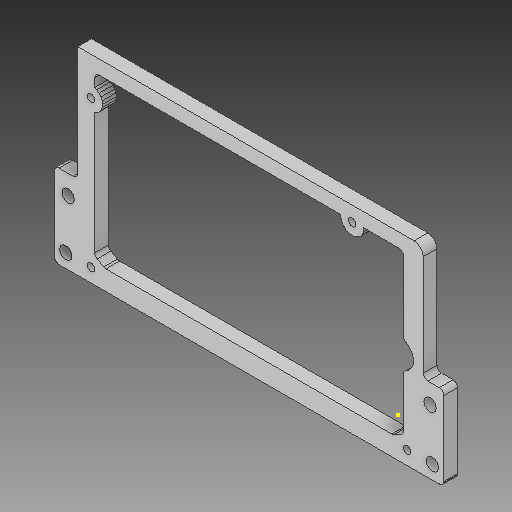
# Autodesk Inventor part: PSU Mount Hipro
Saved by Autodesk Inventor 2018 (Build 220112000, 112)
## iProperties
Created: 2016-07-03
Part Number: PSU Mount Hipro
Material: Generic
Document SubType Name: Modeling
Designer: joshm
Density: 1 g/cm^3
Appearance: Default
Author: joshm
Autodesk Inventor part; units mm, degrees
(part 1 of 2)
ref_plane "YZ Plane" through (0, 0, 0) normal (1, 0, 0) x (0, 1, 0)
ref_plane "XZ Plane" through (0, 0, 0) normal (0, 1, 0) x (-1, 0, 0)
ref_plane "XY Plane" through (0, 0, 0) normal (0, 0, 1) x (1, 0, 0)
sketch "Sketch1" plane through (0, 0, 0) normal (0, 0, 1) x (1, 0, 0)
  line L0 (-149.9319, 87.3176) -> (-150, 86.8)
  line L1 (-150, 86.8) -> (-150, -15.2)
  line L2 (-150, -15.2) -> (-149.9319, -15.7176)
  line L3 (-149.9319, -15.7176) -> (-149.8478, -15.9654)
  line L4 (-149.8478, -15.9654) -> (-149.7321, -16.2)
  line L5 (-149.7321, -16.2) -> (-149.5867, -16.4175)
  line L6 (-149.5867, -16.4175) -> (-149.4142, -16.6142)
  line L7 (-149.4142, -16.6142) -> (-149.2175, -16.7867)
  line L8 (-149.2175, -16.7867) -> (-149, -16.9321)
  line L9 (-149, -16.9321) -> (-148.7654, -17.0478)
  line L10 (-148.7654, -17.0478) -> (-148.5176, -17.1319)
  line L11 (-148.5176, -17.1319) -> (-148, -17.2)
  line L12 (-148, -17.2) -> (18, -17.2)
  line L13 (18, -17.2) -> (18.5176, -17.1319)
  line L14 (18.5176, -17.1319) -> (18.7654, -17.0478)
  line L15 (18.7654, -17.0478) -> (19, -16.9321)
  line L16 (19, -16.9321) -> (19.2175, -16.7867)
  line L17 (19.2175, -16.7867) -> (19.4142, -16.6142)
  line L18 (19.4142, -16.6142) -> (19.5867, -16.4175)
  line L19 (19.5867, -16.4175) -> (19.7321, -16.2)
  line L20 (19.7321, -16.2) -> (19.8478, -15.9654)
  line L21 (19.8478, -15.9654) -> (19.9319, -15.7176)
  line L22 (19.9319, -15.7176) -> (20, -15.2)
  line L23 (20, -15.2) -> (20, 19.2664)
  line L24 (20, 19.2664) -> (11, 19.2664)
  line L25 (11, 19.2664) -> (11, 88.8)
  line L26 (11, 88.8) -> (-148, 88.8)
  line L27 (-148, 88.8) -> (-148.5176, 88.7319)
  line L28 (-148.5176, 88.7319) -> (-148.7654, 88.6478)
  line L29 (-148.7654, 88.6478) -> (-149, 88.5321)
  line L30 (-149, 88.5321) -> (-149.2175, 88.3867)
  line L31 (-149.2175, 88.3867) -> (-149.4142, 88.2142)
  line L32 (-149.4142, 88.2142) -> (-149.5867, 88.0175)
  line L33 (-149.5867, 88.0175) -> (-149.7321, 87.8)
  line L34 (-149.7321, 87.8) -> (-149.8478, 87.5654)
  line L35 (-149.8478, 87.5654) -> (-149.9319, 87.3176)
  line L36 (14.6729, 8.2886) -> (14, 8.2)
  line L37 (14, 8.2) -> (13.3271, 8.2886)
  line L38 (13.3271, 8.2886) -> (12.7, 8.5483)
  line L39 (12.7, 8.5483) -> (12.1615, 8.9615)
  line L40 (12.1615, 8.9615) -> (11.7483, 9.5)
  line L41 (11.7483, 9.5) -> (11.4886, 10.1271)
  line L42 (11.4886, 10.1271) -> (11.4, 10.8)
  line L43 (11.4, 10.8) -> (11.4886, 11.4729)
  line L44 (11.4886, 11.4729) -> (11.7483, 12.1)
  line L45 (11.7483, 12.1) -> (12.1615, 12.6385)
  line L46 (12.1615, 12.6385) -> (12.7, 13.0517)
  line L47 (12.7, 13.0517) -> (13.3271, 13.3114)
  line L48 (13.3271, 13.3114) -> (14, 13.4)
  line L49 (14, 13.4) -> (14.6729, 13.3114)
  line L50 (14.6729, 13.3114) -> (15.3, 13.0517)
  line L51 (15.3, 13.0517) -> (15.8385, 12.6385)
  line L52 (15.8385, 12.6385) -> (16.2517, 12.1)
  line L53 (16.2517, 12.1) -> (16.5114, 11.4729)
  line L54 (16.5114, 11.4729) -> (16.6, 10.8)
  line L55 (16.6, 10.8) -> (16.5114, 10.1271)
  line L56 (16.5114, 10.1271) -> (16.2517, 9.5)
  line L57 (16.2517, 9.5) -> (15.8385, 8.9615)
  line L58 (15.8385, 8.9615) -> (15.3, 8.5483)
  line L59 (15.3, 8.5483) -> (14.6729, 8.2886)
  line L60 (-135.5455, -11.6141) -> (-135.6, -11.2)
  line L61 (-135.6, -11.2) -> (-135.5455, -10.7859)
  line L62 (-135.5455, -10.7859) -> (-135.3856, -10.4)
  line L63 (-135.3856, -10.4) -> (-135.1314, -10.0686)
  line L64 (-135.1314, -10.0686) -> (-134.8, -9.8144)
  line L65 (-134.8, -9.8144) -> (-134.4141, -9.6545)
  line L66 (-134.4141, -9.6545) -> (-134, -9.6)
  line L67 (-134, -9.6) -> (-133.5859, -9.6545)
  line L68 (-133.5859, -9.6545) -> (-133.2, -9.8144)
  line L69 (-133.2, -9.8144) -> (-132.8686, -10.0686)
  line L70 (-132.8686, -10.0686) -> (-132.6144, -10.4)
  line L71 (-132.6144, -10.4) -> (-132.4545, -10.7859)
  line L72 (-132.4545, -10.7859) -> (-132.4, -11.2)
  line L73 (-132.4, -11.2) -> (-132.4545, -11.6141)
  line L74 (-132.4545, -11.6141) -> (-132.6144, -12)
  line L75 (-132.6144, -12) -> (-132.8686, -12.3314)
  line L76 (-132.8686, -12.3314) -> (-133.2, -12.5856)
  line L77 (-133.2, -12.5856) -> (-133.5859, -12.7455)
  line L78 (-133.5859, -12.7455) -> (-134, -12.8)
  line L79 (-134, -12.8) -> (-134.4141, -12.7455)
  line L80 (-134.4141, -12.7455) -> (-134.8, -12.5856)
  line L81 (-134.8, -12.5856) -> (-135.1314, -12.3314)
  line L82 (-135.1314, -12.3314) -> (-135.3856, -12)
  line L83 (-135.3856, -12) -> (-135.5455, -11.6141)
  line L84 (5.6, -11.2) -> (5.5455, -11.6141)
  line L85 (5.5455, -11.6141) -> (5.3856, -12)
  line L86 (5.3856, -12) -> (5.1314, -12.3314)
  line L87 (5.1314, -12.3314) -> (4.8, -12.5856)
  line L88 (4.8, -12.5856) -> (4.4141, -12.7455)
  line L89 (4.4141, -12.7455) -> (4, -12.8)
  line L90 (4, -12.8) -> (3.5859, -12.7455)
  line L91 (3.5859, -12.7455) -> (3.2, -12.5856)
  line L92 (3.2, -12.5856) -> (2.8686, -12.3314)
  line L93 (2.8686, -12.3314) -> (2.6144, -12)
  line L94 (2.6144, -12) -> (2.4545, -11.6141)
  line L95 (2.4545, -11.6141) -> (2.4, -11.2)
  line L96 (2.4, -11.2) -> (2.4545, -10.7859)
  line L97 (2.4545, -10.7859) -> (2.6144, -10.4)
  line L98 (2.6144, -10.4) -> (2.8686, -10.0686)
  line L99 (2.8686, -10.0686) -> (3.2, -9.8144)
  line L100 (3.2, -9.8144) -> (3.5859, -9.6545)
  line L101 (3.5859, -9.6545) -> (4, -9.6)
  line L102 (4, -9.6) -> (4.4141, -9.6545)
  line L103 (4.4141, -9.6545) -> (4.8, -9.8144)
  line L104 (4.8, -9.8144) -> (5.1314, -10.0686)
  line L105 (5.1314, -10.0686) -> (5.3856, -10.4)
  line L106 (5.3856, -10.4) -> (5.5455, -10.7859)
  line L107 (5.5455, -10.7859) -> (5.6, -11.2)
  line L108 (-108.7, 78.5483) -> (-109.3271, 78.2886)
  line L109 (-109.3271, 78.2886) -> (-110, 78.2)
  line L110 (-110, 78.2) -> (-110.6729, 78.2886)
  line L111 (-110.6729, 78.2886) -> (-111.3, 78.5483)
  line L112 (-111.3, 78.5483) -> (-111.8385, 78.9615)
  line L113 (-111.8385, 78.9615) -> (-112.2517, 79.5)
  line L114 (-112.2517, 79.5) -> (-112.5114, 80.1271)
  line L115 (-112.5114, 80.1271) -> (-112.6, 80.8)
  line L116 (-112.6, 80.8) -> (-112.5114, 81.4729)
  line L117 (-112.5114, 81.4729) -> (-112.2517, 82.1)
  line L118 (-112.2517, 82.1) -> (-111.8385, 82.6385)
  line L119 (-111.8385, 82.6385) -> (-111.3, 83.0517)
  line L120 (-111.3, 83.0517) -> (-110.6729, 83.3114)
  line L121 (-110.6729, 83.3114) -> (-110, 83.4)
  line L122 (-110, 83.4) -> (-109.3271, 83.3114)
  line L123 (-109.3271, 83.3114) -> (-108.7, 83.0517)
  line L124 (-108.7, 83.0517) -> (-108.1615, 82.6385)
  line L125 (-108.1615, 82.6385) -> (-107.7483, 82.1)
  line L126 (-107.7483, 82.1) -> (-107.4886, 81.4729)
  line L127 (-107.4886, 81.4729) -> (-107.4, 80.8)
  line L128 (-107.4, 80.8) -> (-107.4886, 80.1271)
  line L129 (-107.4886, 80.1271) -> (-107.7483, 79.5)
  line L130 (-107.7483, 79.5) -> (-108.1615, 78.9615)
  line L131 (-108.1615, 78.9615) -> (-108.7, 78.5483)
  line L132 (-142.8159, -4.2) -> (-142.8159, -7.2)
  line L133 (-142.8159, -7.2) -> (-147.8159, -7.2)
  line L134 (-147.8159, -7.2) -> (-147.8159, -4.2)
  line L135 (-147.8159, -4.2) -> (-142.8159, -4.2)
  line L136 (-18.8686, 61.6686) -> (-19.2, 61.4144)
  line L137 (-19.2, 61.4144) -> (-19.5859, 61.2545)
  line L138 (-19.5859, 61.2545) -> (-20, 61.2)
  line L139 (-20, 61.2) -> (-20.4141, 61.2545)
  line L140 (-20.4141, 61.2545) -> (-20.8, 61.4144)
  line L141 (-20.8, 61.4144) -> (-21.1314, 61.6686)
  line L142 (-21.1314, 61.6686) -> (-21.3856, 62)
  line L143 (-21.3856, 62) -> (-21.5455, 62.3859)
  line L144 (-21.5455, 62.3859) -> (-21.6, 62.8)
  line L145 (-21.6, 62.8) -> (-21.5455, 63.2141)
  line L146 (-21.5455, 63.2141) -> (-21.3856, 63.6)
  line L147 (-21.3856, 63.6) -> (-21.1314, 63.9314)
  line L148 (-21.1314, 63.9314) -> (-20.8, 64.1856)
  line L149 (-20.8, 64.1856) -> (-20.4141, 64.3455)
  line L150 (-20.4141, 64.3455) -> (-20, 64.4)
  line L151 (-20, 64.4) -> (-19.5859, 64.3455)
  line L152 (-19.5859, 64.3455) -> (-19.2, 64.1856)
  line L153 (-19.2, 64.1856) -> (-18.8686, 63.9314)
  line L154 (-18.8686, 63.9314) -> (-18.6144, 63.6)
  line L155 (-18.6144, 63.6) -> (-18.4545, 63.2141)
  line L156 (-18.4545, 63.2141) -> (-18.4, 62.8)
  line L157 (-18.4, 62.8) -> (-18.4545, 62.3859)
  line L158 (-18.4545, 62.3859) -> (-18.6144, 62)
  line L159 (-18.6144, 62) -> (-18.8686, 61.6686)
  line L160 (-20, 78.2) -> (-20.6729, 78.2886)
  line L161 (-20.6729, 78.2886) -> (-21.3, 78.5483)
  line L162 (-21.3, 78.5483) -> (-21.8385, 78.9615)
  line L163 (-21.8385, 78.9615) -> (-22.2517, 79.5)
  line L164 (-22.2517, 79.5) -> (-22.5114, 80.1271)
  line L165 (-22.5114, 80.1271) -> (-22.6, 80.8)
  line L166 (-22.6, 80.8) -> (-22.5114, 81.4729)
  line L167 (-22.5114, 81.4729) -> (-22.2517, 82.1)
  line L168 (-22.2517, 82.1) -> (-21.8385, 82.6385)
  line L169 (-21.8385, 82.6385) -> (-21.3, 83.0517)
  line L170 (-21.3, 83.0517) -> (-20.6729, 83.3114)
  line L171 (-20.6729, 83.3114) -> (-20, 83.4)
  line L172 (-20, 83.4) -> (-19.3271, 83.3114)
  line L173 (-19.3271, 83.3114) -> (-18.7, 83.0517)
  line L174 (-18.7, 83.0517) -> (-18.1615, 82.6385)
  line L175 (-18.1615, 82.6385) -> (-17.7483, 82.1)
  line L176 (-17.7483, 82.1) -> (-17.4886, 81.4729)
  line L177 (-17.4886, 81.4729) -> (-17.4, 80.8)
  line L178 (-17.4, 80.8) -> (-17.4886, 80.1271)
  line L179 (-17.4886, 80.1271) -> (-17.7483, 79.5)
  line L180 (-17.7483, 79.5) -> (-18.1615, 78.9615)
  line L181 (-18.1615, 78.9615) -> (-18.7, 78.5483)
  line L182 (-18.7, 78.5483) -> (-19.3271, 78.2886)
  line L183 (-19.3271, 78.2886) -> (-20, 78.2)
  line L184 (-132.4545, 52.3859) -> (-132.6144, 52)
  line L185 (-132.6144, 52) -> (-132.8686, 51.6686)
  line L186 (-132.8686, 51.6686) -> (-133.2, 51.4144)
  line L187 (-133.2, 51.4144) -> (-133.5859, 51.2545)
  line L188 (-133.5859, 51.2545) -> (-134, 51.2)
  line L189 (-134, 51.2) -> (-134.4141, 51.2545)
  line L190 (-134.4141, 51.2545) -> (-134.8, 51.4144)
  line L191 (-134.8, 51.4144) -> (-135.1314, 51.6686)
  line L192 (-135.1314, 51.6686) -> (-135.3856, 52)
  line L193 (-135.3856, 52) -> (-135.5455, 52.3859)
  line L194 (-135.5455, 52.3859) -> (-135.6, 52.8)
  line L195 (-135.6, 52.8) -> (-135.5455, 53.2141)
  line L196 (-135.5455, 53.2141) -> (-135.3856, 53.6)
  line L197 (-135.3856, 53.6) -> (-135.1314, 53.9314)
  line L198 (-135.1314, 53.9314) -> (-134.8, 54.1856)
  line L199 (-134.8, 54.1856) -> (-134.4141, 54.3455)
  line L200 (-134.4141, 54.3455) -> (-134, 54.4)
  line L201 (-134, 54.4) -> (-133.5859, 54.3455)
  line L202 (-133.5859, 54.3455) -> (-133.2, 54.1856)
  line L203 (-133.2, 54.1856) -> (-132.8686, 53.9314)
  line L204 (-132.8686, 53.9314) -> (-132.6144, 53.6)
  line L205 (-132.6144, 53.6) -> (-132.4545, 53.2141)
  line L206 (-132.4545, 53.2141) -> (-132.4, 52.8)
  line L207 (-132.4, 52.8) -> (-132.4545, 52.3859)
  line L208 (-129.6699, 50.3) -> (-129.1704, 51.5059)
  line L209 (-129.1704, 51.5059) -> (-129, 52.8)
  line L210 (-129, 52.8) -> (-129.1704, 54.0941)
  line L211 (-129.1704, 54.0941) -> (-129.6699, 55.3)
  line L212 (-129.6699, 55.3) -> (-130.4645, 56.3355)
  line L213 (-130.4645, 56.3355) -> (-131.5, 57.1301)
  line L214 (-131.5, 57.1301) -> (-132.4, 57.5029)
  line L215 (-132.4, 57.5029) -> (-132.4, 63.2)
  line L216 (-132.4, 63.2) -> (-24.9458, 63.212)
  line L217 (-24.9458, 63.212) -> (-25, 62.8)
  line L218 (-25, 62.8) -> (-24.8296, 61.5059)
  line L219 (-24.8296, 61.5059) -> (-24.3301, 60.3)
  line L220 (-24.3301, 60.3) -> (-23.5355, 59.2645)
  line L221 (-23.5355, 59.2645) -> (-22.5, 58.4699)
  line L222 (-22.5, 58.4699) -> (-21.2941, 57.9704)
  line L223 (-21.2941, 57.9704) -> (-20, 57.8)
  line L224 (-20, 57.8) -> (-18.7059, 57.9704)
  line L225 (-18.7059, 57.9704) -> (-17.5, 58.4699)
  line L226 (-17.5, 58.4699) -> (-16.4645, 59.2645)
  line L227 (-16.4645, 59.2645) -> (-15.6699, 60.3)
  line L228 (-15.6699, 60.3) -> (-15.1704, 61.5059)
  line L229 (-15.1704, 61.5059) -> (-15, 62.8)
  line L230 (-15, 62.8) -> (-15.0542, 63.2118)
  line L231 (-15.0542, 63.2118) -> (2.4, 63.2)
  line L232 (2.4, 63.2) -> (2.4, -6.2)
  line L233 (2.4, -6.2) -> (-2.1698, -8.6089)
  line L234 (-2.1698, -8.6089) -> (-128.0185, -8.6089)
  line L235 (-128.0185, -8.6089) -> (-132.4, -6.2)
  line L236 (-132.4, -6.2) -> (-132.4, 48.0971)
  line L237 (-132.4, 48.0971) -> (-131.5, 48.4699)
  line L238 (-131.5, 48.4699) -> (-130.4645, 49.2645)
  line L239 (-130.4645, 49.2645) -> (-129.6699, 50.3)
  line L240 (-142.392, -10.5012) -> (-142.3, -11.2)
  line L241 (-142.3, -11.2) -> (-142.392, -11.8988)
  line L242 (-142.392, -11.8988) -> (-142.6617, -12.55)
  line L243 (-142.6617, -12.55) -> (-143.0908, -13.1092)
  line L244 (-143.0908, -13.1092) -> (-143.65, -13.5383)
  line L245 (-143.65, -13.5383) -> (-144.3012, -13.808)
  line L246 (-144.3012, -13.808) -> (-145, -13.9)
  line L247 (-145, -13.9) -> (-145.6988, -13.808)
  line L248 (-145.6988, -13.808) -> (-146.35, -13.5383)
  line L249 (-146.35, -13.5383) -> (-146.9092, -13.1092)
  line L250 (-146.9092, -13.1092) -> (-147.3383, -12.55)
  line L251 (-147.3383, -12.55) -> (-147.608, -11.8988)
  line L252 (-147.608, -11.8988) -> (-147.7, -11.2)
  line L253 (-147.7, -11.2) -> (-147.608, -10.5012)
  line L254 (-147.608, -10.5012) -> (-147.3383, -9.85)
  line L255 (-147.3383, -9.85) -> (-146.9092, -9.2908)
  line L256 (-146.9092, -9.2908) -> (-146.35, -8.8617)
  line L257 (-146.35, -8.8617) -> (-145.6988, -8.592)
  line L258 (-145.6988, -8.592) -> (-145, -8.5)
  line L259 (-145, -8.5) -> (-144.3012, -8.592)
  line L260 (-144.3012, -8.592) -> (-143.65, -8.8617)
  line L261 (-143.65, -8.8617) -> (-143.0908, -9.2908)
  line L262 (-143.0908, -9.2908) -> (-142.6617, -9.85)
  line L263 (-142.6617, -9.85) -> (-142.392, -10.5012)
  line L264 (12.3, -11.2) -> (12.392, -10.5012)
  line L265 (12.392, -10.5012) -> (12.6617, -9.85)
  line L266 (12.6617, -9.85) -> (13.0908, -9.2908)
  line L267 (13.0908, -9.2908) -> (13.65, -8.8617)
  line L268 (13.65, -8.8617) -> (14.3012, -8.592)
  line L269 (14.3012, -8.592) -> (15, -8.5)
  line L270 (15, -8.5) -> (15.6988, -8.592)
  line L271 (15.6988, -8.592) -> (16.35, -8.8617)
  line L272 (16.35, -8.8617) -> (16.9092, -9.2908)
  line L273 (16.9092, -9.2908) -> (17.3383, -9.85)
  line L274 (17.3383, -9.85) -> (17.608, -10.5012)
  line L275 (17.608, -10.5012) -> (17.7, -11.2)
  line L276 (17.7, -11.2) -> (17.608, -11.8988)
  line L277 (17.608, -11.8988) -> (17.3383, -12.55)
  line L278 (17.3383, -12.55) -> (16.9092, -13.1092)
  line L279 (16.9092, -13.1092) -> (16.35, -13.5383)
  line L280 (16.35, -13.5383) -> (15.6988, -13.808)
  line L281 (15.6988, -13.808) -> (15, -13.9)
  line L282 (15, -13.9) -> (14.3012, -13.808)
  line L283 (14.3012, -13.808) -> (13.65, -13.5383)
  line L284 (13.65, -13.5383) -> (13.0908, -13.1092)
  line L285 (13.0908, -13.1092) -> (12.6617, -12.55)
  line L286 (12.6617, -12.55) -> (12.392, -11.8988)
  line L287 (12.392, -11.8988) -> (12.3, -11.2)
  line L288 (-142.392, 59.4988) -> (-142.3, 58.8)
  line L289 (-142.3, 58.8) -> (-142.392, 58.1012)
  line L290 (-142.392, 58.1012) -> (-142.6617, 57.45)
  line L291 (-142.6617, 57.45) -> (-143.0908, 56.8908)
  line L292 (-143.0908, 56.8908) -> (-143.65, 56.4617)
  line L293 (-143.65, 56.4617) -> (-144.3012, 56.192)
  line L294 (-144.3012, 56.192) -> (-145, 56.1)
  line L295 (-145, 56.1) -> (-145.6988, 56.192)
  line L296 (-145.6988, 56.192) -> (-146.35, 56.4617)
  line L297 (-146.35, 56.4617) -> (-146.9092, 56.8908)
  line L298 (-146.9092, 56.8908) -> (-147.3383, 57.45)
  line L299 (-147.3383, 57.45) -> (-147.608, 58.1012)
  line L300 (-147.608, 58.1012) -> (-147.7, 58.8)
  line L301 (-147.7, 58.8) -> (-147.608, 59.4988)
  line L302 (-147.608, 59.4988) -> (-147.3383, 60.15)
  line L303 (-147.3383, 60.15) -> (-146.9092, 60.7092)
  line L304 (-146.9092, 60.7092) -> (-146.35, 61.1383)
  line L305 (-146.35, 61.1383) -> (-145.6988, 61.408)
  line L306 (-145.6988, 61.408) -> (-145, 61.5)
  line L307 (-145, 61.5) -> (-144.3012, 61.408)
  line L308 (-144.3012, 61.408) -> (-143.65, 61.1383)
  line L309 (-143.65, 61.1383) -> (-143.0908, 60.7092)
  line L310 (-143.0908, 60.7092) -> (-142.6617, 60.15)
  line L311 (-142.6617, 60.15) -> (-142.392, 59.4988)
  line L312 (-142.1615, 8.9615) -> (-142.3, 8.8553)
  line L313 (-142.3, 8.8553) -> (-142.7, 8.5483)
  line L314 (-142.7, 8.5483) -> (-143.3271, 8.2886)
  line L315 (-143.3271, 8.2886) -> (-144, 8.2)
  line L316 (-144, 8.2) -> (-144.6729, 8.2886)
  line L317 (-144.6729, 8.2886) -> (-145.3, 8.5483)
  line L318 (-145.3, 8.5483) -> (-145.8385, 8.9615)
  line L319 (-145.8385, 8.9615) -> (-146.2517, 9.5)
  line L320 (-146.2517, 9.5) -> (-146.5114, 10.1271)
  line L321 (-146.5114, 10.1271) -> (-146.6, 10.8)
  line L322 (-146.6, 10.8) -> (-146.5114, 11.4729)
  line L323 (-146.5114, 11.4729) -> (-146.2517, 12.1)
  line L324 (-146.2517, 12.1) -> (-145.8385, 12.6385)
  line L325 (-145.8385, 12.6385) -> (-145.3, 13.0517)
  line L326 (-145.3, 13.0517) -> (-144.6729, 13.3114)
  line L327 (-144.6729, 13.3114) -> (-144, 13.4)
  line L328 (-144, 13.4) -> (-143.3271, 13.3114)
  line L329 (-143.3271, 13.3114) -> (-142.7, 13.0517)
  line L330 (-142.7, 13.0517) -> (-142.3, 12.7447)
  line L331 (-142.3, 12.7447) -> (-142.1615, 12.6385)
  line L332 (-142.1615, 12.6385) -> (-141.7483, 12.1)
  line L333 (-141.7483, 12.1) -> (-141.4886, 11.4729)
  line L334 (-141.4886, 11.4729) -> (-141.4, 10.8)
  line L335 (-141.4, 10.8) -> (-141.4886, 10.1271)
  line L336 (-141.4886, 10.1271) -> (-141.7483, 9.5)
  line L337 (-141.7483, 9.5) -> (-142.1615, 8.9615)
  point P0 (0, 0)
  constraints: 676 end point
extrude "Extrusion1" add sketch "Sketch1" along normal blind 6
sketch "Sketch2" plane through (0, 0, 6) normal (0, 0, 1) x (1, 0, 0)
  line L0 (11, 19.2664) -> (11, 88.8) projected
  line L1 (11, 19.2664) -> (11, 24.0664)
  line L2 (11, 19.2664) -> (15.8, 19.2664) construction
  circle A0 centre (11, 24.0664) radius 3
  point P0 (0, 0)
  dimension "d3" = 90
  constraints: 4 end point, 1 centre point, 1 coincident, 1 collinear, 1 horizontal, 1 perpendicular
  measures "d3" angle of L2 L1
extrude "Extrusion2" cut sketch "Sketch2" against normal blind 6
fillet "Fillet1" radius 2 3 edges at (11, 19.2664, 3) (11, 27.0664, 3) (11, 21.0664, 3)
fillet "Fillet2" radius 2 1 edges at (11, 88.8, 3)
fillet "Fillet3" radius 2 3 edges at (-132.4, 63.2, 3) (-132.4, -6.2, 3) (-128.0185, -8.6089, 3)
fillet "Fillet4" radius 2 3 edges at (2.4, 63.2, 3) (-2.1698, -8.6089, 3) (2.4, -6.2, 3)
fillet "Fillet5" radius 2 1 edges at (20, 19.2664, 3)
sketch "Sketch3" plane through (0, 0, 6) normal (0, 0, 1) x (1, 0, 0)
  arc A0 (20, 17.2664) -> (18, 19.2664) centre (18, 17.2664) ccw
  line L0 (18, 19.2664) -> (12.5808, 19.2664)
  arc A1 (10.7904, 20.3751) -> (12.5808, 19.2664) centre (12.5808, 21.2664) ccw
  arc A2 (10.7904, 20.3751) -> (9.8, 21.3169) centre (9, 19.4838) ccw
  arc A3 (9.8, 26.816) -> (9.8, 21.3169) centre (11, 24.0664) ccw
  arc A4 (9.8, 26.816) -> (11, 28.649) centre (9, 28.649) ccw
  line L1 (11, 28.649) -> (11, 86.8) projected
  arc A5 (9, 88.8) -> (11, 86.8) centre (9, 86.8) ccw projected
  line L2 (9, 88.8) -> (-148, 88.8) projected
  line L3 (-148, 88.8) -> (-148.5176, 88.7319) projected
  line L4 (-148.5176, 88.7319) -> (-148.7654, 88.6478) projected
  line L5 (-148.7654, 88.6478) -> (-149, 88.5321) projected
  line L6 (-149, 88.5321) -> (-149.2175, 88.3867) projected
  line L7 (-149.2175, 88.3867) -> (-149.4142, 88.2142) projected
  line L8 (-149.4142, 88.2142) -> (-149.5867, 88.0175) projected
  line L9 (-149.5867, 88.0175) -> (-149.7321, 87.8) projected
  line L10 (-149.7321, 87.8) -> (-149.8478, 87.5654) projected
  line L11 (-149.8478, 87.5654) -> (-149.9319, 87.3176) projected
  line L12 (-149.9319, 87.3176) -> (-150, 86.8) projected
  line L13 (-150, 86.8) -> (-150, -15.2) projected
  line L14 (-150, -15.2) -> (-149.9319, -15.7176) projected
  line L15 (-149.9319, -15.7176) -> (-149.8478, -15.9654) projected
  line L16 (-149.8478, -15.9654) -> (-149.7321, -16.2) projected
  line L17 (-149.7321, -16.2) -> (-149.5867, -16.4175) projected
  line L18 (-149.5867, -16.4175) -> (-149.4142, -16.6142) projected
  line L19 (-149.4142, -16.6142) -> (-149.2175, -16.7867) projected
  line L20 (-149.2175, -16.7867) -> (-149, -16.9321) projected
  line L21 (-149, -16.9321) -> (-148.7654, -17.0478) projected
  line L22 (-148.7654, -17.0478) -> (-148.5176, -17.1319) projected
  line L23 (-148.5176, -17.1319) -> (-148, -17.2) projected
  line L24 (-148, -17.2) -> (18, -17.2) projected
  line L25 (18, -17.2) -> (18.5176, -17.1319) projected
  line L26 (18.5176, -17.1319) -> (18.7654, -17.0478) projected
  line L27 (18.7654, -17.0478) -> (19, -16.9321) projected
  line L28 (19, -16.9321) -> (19.2175, -16.7867) projected
  line L29 (19.2175, -16.7867) -> (19.4142, -16.6142) projected
  line L30 (19.4142, -16.6142) -> (19.5867, -16.4175) projected
  line L31 (19.5867, -16.4175) -> (19.7321, -16.2) projected
  line L32 (19.7321, -16.2) -> (19.8478, -15.9654) projected
  line L33 (19.8478, -15.9654) -> (19.9319, -15.7176) projected
  line L34 (19.9319, -15.7176) -> (20, -15.2) projected
  line L35 (20, -15.2) -> (20, 17.2664) projected
  line L36 (-129, 52.8) -> (-129.1704, 54.0941) projected
  line L37 (-129.1704, 54.0941) -> (-129.6699, 55.3) projected
  line L38 (-129.6699, 55.3) -> (-130.4645, 56.3355) projected
  line L39 (-130.4645, 56.3355) -> (-131.5, 57.1301) projected
  line L40 (-131.5, 57.1301) -> (-132.4, 57.5029) projected
  line L41 (-132.4, 57.5029) -> (-132.4, 61.2002) projected
  arc A6 (-130.4002, 63.2002) -> (-132.4, 61.2002) centre (-130.4, 61.2002) ccw projected
  line L42 (-130.4002, 63.2002) -> (-24.9458, 63.212) projected
  line L43 (-24.9458, 63.212) -> (-25, 62.8) projected
  line L44 (-25, 62.8) -> (-24.8296, 61.5059) projected
  line L45 (-24.8296, 61.5059) -> (-24.3301, 60.3) projected
  line L46 (-24.3301, 60.3) -> (-23.5355, 59.2645) projected
  line L47 (-23.5355, 59.2645) -> (-22.5, 58.4699) projected
  line L48 (-22.5, 58.4699) -> (-21.2941, 57.9704) projected
  line L49 (-21.2941, 57.9704) -> (-20, 57.8) projected
  line L50 (-20, 57.8) -> (-18.7059, 57.9704) projected
  line L51 (-18.7059, 57.9704) -> (-17.5, 58.4699) projected
  line L52 (-17.5, 58.4699) -> (-16.4645, 59.2645) projected
  line L53 (-16.4645, 59.2645) -> (-15.6699, 60.3) projected
  line L54 (-15.6699, 60.3) -> (-15.1704, 61.5059) projected
  line L55 (-15.1704, 61.5059) -> (-15, 62.8) projected
  line L56 (-15, 62.8) -> (-15.0542, 63.2118) projected
  line L57 (-15.0542, 63.2118) -> (0.4014, 63.2014) projected
  arc A7 (2.4, 61.2014) -> (0.4014, 63.2014) centre (0.4, 61.2014) ccw projected
  line L58 (2.4, 61.2014) -> (2.4, -4.9934) projected
  arc A8 (1.3326, -6.7626) -> (2.4, -4.9934) centre (0.4, -4.9934) ccw projected
  line L59 (1.3326, -6.7626) -> (-1.7321, -8.3782) projected
  arc A9 (-2.6647, -8.6089) -> (-1.7321, -8.3782) centre (-2.6647, -6.6089) ccw projected
  line L60 (-2.6647, -8.6089) -> (-127.505, -8.6089) projected
  arc A10 (-128.4686, -8.3615) -> (-127.505, -8.6089) centre (-127.505, -6.6089) ccw projected
  line L61 (-128.4686, -8.3615) -> (-131.3636, -6.7698) projected
  arc A11 (-132.4, -5.0172) -> (-131.3636, -6.7698) centre (-130.4, -5.0172) ccw projected
  line L62 (-132.4, -5.0172) -> (-132.4, 48.0971) projected
  line L63 (-132.4, 48.0971) -> (-131.5, 48.4699) projected
  line L64 (-131.5, 48.4699) -> (-130.4645, 49.2645) projected
  line L65 (-130.4645, 49.2645) -> (-129.6699, 50.3) projected
  line L66 (-129.6699, 50.3) -> (-129.1704, 51.5059) projected
  line L67 (-129.1704, 51.5059) -> (-129, 52.8) projected
  line L68 (-142.392, 58.1012) -> (-142.6617, 57.45) projected
  line L69 (-142.6617, 57.45) -> (-143.0908, 56.8908) projected
  line L70 (-143.0908, 56.8908) -> (-143.65, 56.4617) projected
  line L71 (-143.65, 56.4617) -> (-144.3012, 56.192) projected
  line L72 (-144.3012, 56.192) -> (-145, 56.1) projected
  line L73 (-145, 56.1) -> (-145.6988, 56.192) projected
  line L74 (-145.6988, 56.192) -> (-146.35, 56.4617) projected
  line L75 (-146.35, 56.4617) -> (-146.9092, 56.8908) projected
  line L76 (-146.9092, 56.8908) -> (-147.3383, 57.45) projected
  line L77 (-147.3383, 57.45) -> (-147.608, 58.1012) projected
  line L78 (-147.608, 58.1012) -> (-147.7, 58.8) projected
  line L79 (-147.7, 58.8) -> (-147.608, 59.4988) projected
  line L80 (-147.608, 59.4988) -> (-147.3383, 60.15) projected
  line L81 (-147.3383, 60.15) -> (-146.9092, 60.7092) projected
  line L82 (-146.9092, 60.7092) -> (-146.35, 61.1383) projected
  line L83 (-146.35, 61.1383) -> (-145.6988, 61.408) projected
  line L84 (-145.6988, 61.408) -> (-145, 61.5) projected
  line L85 (-145, 61.5) -> (-144.3012, 61.408) projected
  line L86 (-144.3012, 61.408) -> (-143.65, 61.1383) projected
  line L87 (-143.65, 61.1383) -> (-143.0908, 60.7092) projected
  line L88 (-143.0908, 60.7092) -> (-142.6617, 60.15) projected
  line L89 (-142.6617, 60.15) -> (-142.392, 59.4988) projected
  line L90 (-142.392, 59.4988) -> (-142.3, 58.8) projected
  line L91 (-142.3, 58.8) -> (-142.392, 58.1012) projected
  line L92 (12.6617, -9.85) -> (13.0908, -9.2908) projected
  line L93 (13.0908, -9.2908) -> (13.65, -8.8617) projected
  line L94 (13.65, -8.8617) -> (14.3012, -8.592) projected
  line L95 (14.3012, -8.592) -> (15, -8.5) projected
  line L96 (15, -8.5) -> (15.6988, -8.592) projected
  line L97 (15.6988, -8.592) -> (16.35, -8.8617) projected
  line L98 (16.35, -8.8617) -> (16.9092, -9.2908) projected
  line L99 (16.9092, -9.2908) -> (17.3383, -9.85) projected
  line L100 (17.3383, -9.85) -> (17.608, -10.5012) projected
  line L101 (17.608, -10.5012) -> (17.7, -11.2) projected
  line L102 (17.7, -11.2) -> (17.608, -11.8988) projected
  line L103 (17.608, -11.8988) -> (17.3383, -12.55) projected
  line L104 (17.3383, -12.55) -> (16.9092, -13.1092) projected
  line L105 (16.9092, -13.1092) -> (16.35, -13.5383) projected
  line L106 (16.35, -13.5383) -> (15.6988, -13.808) projected
  line L107 (15.6988, -13.808) -> (15, -13.9) projected
  line L108 (15, -13.9) -> (14.3012, -13.808) projected
  line L109 (14.3012, -13.808) -> (13.65, -13.5383) projected
  line L110 (13.65, -13.5383) -> (13.0908, -13.1092) projected
  line L111 (13.0908, -13.1092) -> (12.6617, -12.55) projected
  line L112 (12.6617, -12.55) -> (12.392, -11.8988) projected
  line L113 (12.392, -11.8988) -> (12.3, -11.2) projected
  line L114 (12.3, -11.2) -> (12.392, -10.5012) projected
  line L115 (12.392, -10.5012) -> (12.6617, -9.85) projected
  line L116 (-142.392, -11.8988) -> (-142.6617, -12.55) projected
  line L117 (-142.6617, -12.55) -> (-143.0908, -13.1092) projected
  line L118 (-143.0908, -13.1092) -> (-143.65, -13.5383) projected
  line L119 (-143.65, -13.5383) -> (-144.3012, -13.808) projected
  line L120 (-144.3012, -13.808) -> (-145, -13.9) projected
  line L121 (-145, -13.9) -> (-145.6988, -13.808) projected
  line L122 (-145.6988, -13.808) -> (-146.35, -13.5383) projected
  line L123 (-146.35, -13.5383) -> (-146.9092, -13.1092) projected
  line L124 (-146.9092, -13.1092) -> (-147.3383, -12.55) projected
  line L125 (-147.3383, -12.55) -> (-147.608, -11.8988) projected
  line L126 (-147.608, -11.8988) -> (-147.7, -11.2) projected
  line L127 (-147.7, -11.2) -> (-147.608, -10.5012) projected
  line L128 (-147.608, -10.5012) -> (-147.3383, -9.85) projected
  line L129 (-147.3383, -9.85) -> (-146.9092, -9.2908) projected
  line L130 (-146.9092, -9.2908) -> (-146.35, -8.8617) projected
  line L131 (-146.35, -8.8617) -> (-145.6988, -8.592) projected
  line L132 (-145.6988, -8.592) -> (-145, -8.5) projected
  line L133 (-145, -8.5) -> (-144.3012, -8.592) projected
  line L134 (-144.3012, -8.592) -> (-143.65, -8.8617) projected
  line L135 (-143.65, -8.8617) -> (-143.0908, -9.2908) projected
  line L136 (-143.0908, -9.2908) -> (-142.6617, -9.85) projected
  line L137 (-142.6617, -9.85) -> (-142.392, -10.5012) projected
  line L138 (-142.392, -10.5012) -> (-142.3, -11.2) projected
  line L139 (-142.3, -11.2) -> (-142.392, -11.8988) projected
  line L140 (-142.7, 8.5483) -> (-143.3271, 8.2886) projected
  line L141 (-143.3271, 8.2886) -> (-144, 8.2) projected
  line L142 (-144, 8.2) -> (-144.6729, 8.2886) projected
  line L143 (-144.6729, 8.2886) -> (-145.3, 8.5483) projected
  line L144 (-145.3, 8.5483) -> (-145.8385, 8.9615) projected
  line L145 (-145.8385, 8.9615) -> (-146.2517, 9.5) projected
  line L146 (-146.2517, 9.5) -> (-146.5114, 10.1271) projected
  line L147 (-146.5114, 10.1271) -> (-146.6, 10.8) projected
  line L148 (-146.6, 10.8) -> (-146.5114, 11.4729) projected
  line L149 (-146.5114, 11.4729) -> (-146.2517, 12.1) projected
  line L150 (-146.2517, 12.1) -> (-145.8385, 12.6385) projected
  line L151 (-145.8385, 12.6385) -> (-145.3, 13.0517) projected
  line L152 (-145.3, 13.0517) -> (-144.6729, 13.3114) projected
  line L153 (-144.6729, 13.3114) -> (-144, 13.4) projected
  line L154 (-144, 13.4) -> (-143.3271, 13.3114) projected
  line L155 (-143.3271, 13.3114) -> (-142.7, 13.0517) projected
  line L156 (-142.7, 13.0517) -> (-142.1615, 12.6385) projected
  line L157 (-142.1615, 12.6385) -> (-141.7483, 12.1) projected
  line L158 (-141.7483, 12.1) -> (-141.4886, 11.4729) projected
  line L159 (-141.4886, 11.4729) -> (-141.4, 10.8) projected
  line L160 (-141.4, 10.8) -> (-141.4886, 10.1271) projected
  line L161 (-141.4886, 10.1271) -> (-141.7483, 9.5) projected
  line L162 (-141.7483, 9.5) -> (-142.1615, 8.9615) projected
  line L163 (-142.1615, 8.9615) -> (-142.7, 8.5483) projected
  line L164 (-21.3, 78.5483) -> (-21.8385, 78.9615) projected
  line L165 (-21.8385, 78.9615) -> (-22.2517, 79.5) projected
  line L166 (-22.2517, 79.5) -> (-22.5114, 80.1271) projected
  line L167 (-22.5114, 80.1271) -> (-22.6, 80.8) projected
  line L168 (-22.6, 80.8) -> (-22.5114, 81.4729) projected
  line L169 (-22.5114, 81.4729) -> (-22.2517, 82.1) projected
  line L170 (-22.2517, 82.1) -> (-21.8385, 82.6385) projected
  line L171 (-21.8385, 82.6385) -> (-21.3, 83.0517) projected
  line L172 (-21.3, 83.0517) -> (-20.6729, 83.3114) projected
  line L173 (-20.6729, 83.3114) -> (-20, 83.4) projected
  line L174 (-20, 83.4) -> (-19.3271, 83.3114) projected
  line L175 (-19.3271, 83.3114) -> (-18.7, 83.0517) projected
  line L176 (-18.7, 83.0517) -> (-18.1615, 82.6385) projected
  line L177 (-18.1615, 82.6385) -> (-17.7483, 82.1) projected
  line L178 (-17.7483, 82.1) -> (-17.4886, 81.4729) projected
  line L179 (-17.4886, 81.4729) -> (-17.4, 80.8) projected
  line L180 (-17.4, 80.8) -> (-17.4886, 80.1271) projected
  line L181 (-17.4886, 80.1271) -> (-17.7483, 79.5) projected
  line L182 (-17.7483, 79.5) -> (-18.1615, 78.9615) projected
  line L183 (-18.1615, 78.9615) -> (-18.7, 78.5483) projected
  line L184 (-18.7, 78.5483) -> (-19.3271, 78.2886) projected
  line L185 (-19.3271, 78.2886) -> (-20, 78.2) projected
  line L186 (-20, 78.2) -> (-20.6729, 78.2886) projected
  line L187 (-20.6729, 78.2886) -> (-21.3, 78.5483) projected
  line L188 (-110, 78.2) -> (-110.6729, 78.2886) projected
  line L189 (-110.6729, 78.2886) -> (-111.3, 78.5483) projected
  line L190 (-111.3, 78.5483) -> (-111.8385, 78.9615) projected
  line L191 (-111.8385, 78.9615) -> (-112.2517, 79.5) projected
  line L192 (-112.2517, 79.5) -> (-112.5114, 80.1271) projected
  line L193 (-112.5114, 80.1271) -> (-112.6, 80.8) projected
  line L194 (-112.6, 80.8) -> (-112.5114, 81.4729) projected
  line L195 (-112.5114, 81.4729) -> (-112.2517, 82.1) projected
  line L196 (-112.2517, 82.1) -> (-111.8385, 82.6385) projected
  line L197 (-111.8385, 82.6385) -> (-111.3, 83.0517) projected
  line L198 (-111.3, 83.0517) -> (-110.6729, 83.3114) projected
  line L199 (-110.6729, 83.3114) -> (-110, 83.4) projected
  line L200 (-110, 83.4) -> (-109.3271, 83.3114) projected
  line L201 (-109.3271, 83.3114) -> (-108.7, 83.0517) projected
  line L202 (-108.7, 83.0517) -> (-108.1615, 82.6385) projected
  line L203 (-108.1615, 82.6385) -> (-107.7483, 82.1) projected
  line L204 (-107.7483, 82.1) -> (-107.4886, 81.4729) projected
  line L205 (-107.4886, 81.4729) -> (-107.4, 80.8) projected
  line L206 (-107.4, 80.8) -> (-107.4886, 80.1271) projected
  line L207 (-107.4886, 80.1271) -> (-107.7483, 79.5) projected
  line L208 (-107.7483, 79.5) -> (-108.1615, 78.9615) projected
  line L209 (-108.1615, 78.9615) -> (-108.7, 78.5483) projected
  line L210 (-108.7, 78.5483) -> (-109.3271, 78.2886) projected
  line L211 (-109.3271, 78.2886) -> (-110, 78.2) projected
  line L212 (13.3271, 8.2886) -> (12.7, 8.5483)
  line L213 (12.7, 8.5483) -> (12.1615, 8.9615)
  line L214 (12.1615, 8.9615) -> (11.7483, 9.5)
  line L215 (11.7483, 9.5) -> (11.4886, 10.1271)
  line L216 (11.4886, 10.1271) -> (11.4, 10.8)
  line L217 (11.4, 10.8) -> (11.4886, 11.4729)
  line L218 (11.4886, 11.4729) -> (11.7483, 12.1)
  line L219 (11.7483, 12.1) -> (12.1615, 12.6385)
  line L220 (12.1615, 12.6385) -> (12.7, 13.0517)
  line L221 (12.7, 13.0517) -> (13.3271, 13.3114)
  line L222 (13.3271, 13.3114) -> (14, 13.4)
  line L223 (14, 13.4) -> (14.6729, 13.3114)
  line L224 (14.6729, 13.3114) -> (15.3, 13.0517)
  line L225 (15.3, 13.0517) -> (15.8385, 12.6385)
  line L226 (15.8385, 12.6385) -> (16.2517, 12.1)
  line L227 (16.2517, 12.1) -> (16.5114, 11.4729)
  line L228 (16.5114, 11.4729) -> (16.6, 10.8)
  line L229 (16.6, 10.8) -> (16.5114, 10.1271)
  line L230 (16.5114, 10.1271) -> (16.2517, 9.5)
  line L231 (16.2517, 9.5) -> (15.8385, 8.9615)
  line L232 (15.8385, 8.9615) -> (15.3, 8.5483)
  line L233 (15.3, 8.5483) -> (14.6729, 8.2886)
  line L234 (14.6729, 8.2886) -> (14, 8.2)
  line L235 (14, 8.2) -> (13.3271, 8.2886)
  line L236 (-147.8159, -7.2) -> (-147.8159, -4.2) projected
  line L237 (-147.8159, -4.2) -> (-142.8159, -4.2) projected
  line L238 (-142.8159, -4.2) -> (-142.8159, -7.2) projected
  line L239 (-142.8159, -7.2) -> (-147.8159, -7.2) projected
  line L240 (-132.8686, 51.6686) -> (-133.2, 51.4144) projected
  line L241 (-133.2, 51.4144) -> (-133.5859, 51.2545) projected
  line L242 (-133.5859, 51.2545) -> (-134, 51.2) projected
  line L243 (-134, 51.2) -> (-134.4141, 51.2545) projected
  line L244 (-134.4141, 51.2545) -> (-134.8, 51.4144) projected
  line L245 (-134.8, 51.4144) -> (-135.1314, 51.6686) projected
  line L246 (-135.1314, 51.6686) -> (-135.3856, 52) projected
  line L247 (-135.3856, 52) -> (-135.5455, 52.3859) projected
  line L248 (-135.5455, 52.3859) -> (-135.6, 52.8) projected
  line L249 (-135.6, 52.8) -> (-135.5455, 53.2141) projected
  line L250 (-135.5455, 53.2141) -> (-135.3856, 53.6) projected
  line L251 (-135.3856, 53.6) -> (-135.1314, 53.9314) projected
  line L252 (-135.1314, 53.9314) -> (-134.8, 54.1856) projected
  line L253 (-134.8, 54.1856) -> (-134.4141, 54.3455) projected
  line L254 (-134.4141, 54.3455) -> (-134, 54.4) projected
  line L255 (-134, 54.4) -> (-133.5859, 54.3455) projected
  line L256 (-133.5859, 54.3455) -> (-133.2, 54.1856) projected
  line L257 (-133.2, 54.1856) -> (-132.8686, 53.9314) projected
  line L258 (-132.8686, 53.9314) -> (-132.6144, 53.6) projected
  line L259 (-132.6144, 53.6) -> (-132.4545, 53.2141) projected
  line L260 (-132.4545, 53.2141) -> (-132.4, 52.8) projected
  line L261 (-132.4, 52.8) -> (-132.4545, 52.3859) projected
  line L262 (-132.4545, 52.3859) -> (-132.6144, 52) projected
  line L263 (-132.6144, 52) -> (-132.8686, 51.6686) projected
  line L264 (-19.5859, 61.2545) -> (-20, 61.2) projected
  line L265 (-20, 61.2) -> (-20.4141, 61.2545) projected
  line L266 (-20.4141, 61.2545) -> (-20.8, 61.4144) projected
  line L267 (-20.8, 61.4144) -> (-21.1314, 61.6686) projected
  line L268 (-21.1314, 61.6686) -> (-21.3856, 62) projected
  line L269 (-21.3856, 62) -> (-21.5455, 62.3859) projected
  line L270 (-21.5455, 62.3859) -> (-21.6, 62.8) projected
  line L271 (-21.6, 62.8) -> (-21.5455, 63.2141) projected
  line L272 (-21.5455, 63.2141) -> (-21.3856, 63.6) projected
  line L273 (-21.3856, 63.6) -> (-21.1314, 63.9314) projected
  line L274 (-21.1314, 63.9314) -> (-20.8, 64.1856) projected
  line L275 (-20.8, 64.1856) -> (-20.4141, 64.3455) projected
  line L276 (-20.4141, 64.3455) -> (-20, 64.4) projected
  line L277 (-20, 64.4) -> (-19.5859, 64.3455) projected
  line L278 (-19.5859, 64.3455) -> (-19.2, 64.1856) projected
  line L279 (-19.2, 64.1856) -> (-18.8686, 63.9314) projected
  line L280 (-18.8686, 63.9314) -> (-18.6144, 63.6) projected
  line L281 (-18.6144, 63.6) -> (-18.4545, 63.2141) projected
  line L282 (-18.4545, 63.2141) -> (-18.4, 62.8) projected
  line L283 (-18.4, 62.8) -> (-18.4545, 62.3859) projected
  line L284 (-18.4545, 62.3859) -> (-18.6144, 62) projected
  line L285 (-18.6144, 62) -> (-18.8686, 61.6686) projected
  line L286 (-18.8686, 61.6686) -> (-19.2, 61.4144) projected
  line L287 (-19.2, 61.4144) -> (-19.5859, 61.2545) projected
  line L288 (5.3856, -12) -> (5.1314, -12.3314) projected
  line L289 (5.1314, -12.3314) -> (4.8, -12.5856) projected
  line L290 (4.8, -12.5856) -> (4.4141, -12.7455) projected
  line L291 (4.4141, -12.7455) -> (4, -12.8) projected
  line L292 (4, -12.8) -> (3.5859, -12.7455) projected
  line L293 (3.5859, -12.7455) -> (3.2, -12.5856) projected
  line L294 (3.2, -12.5856) -> (2.8686, -12.3314) projected
  line L295 (2.8686, -12.3314) -> (2.6144, -12) projected
  line L296 (2.6144, -12) -> (2.4545, -11.6141) projected
  line L297 (2.4545, -11.6141) -> (2.4, -11.2) projected
  line L298 (2.4, -11.2) -> (2.4545, -10.7859) projected
  line L299 (2.4545, -10.7859) -> (2.6144, -10.4) projected
  line L300 (2.6144, -10.4) -> (2.8686, -10.0686) projected
  line L301 (2.8686, -10.0686) -> (3.2, -9.8144) projected
  line L302 (3.2, -9.8144) -> (3.5859, -9.6545) projected
  line L303 (3.5859, -9.6545) -> (4, -9.6) projected
  line L304 (4, -9.6) -> (4.4141, -9.6545) projected
  line L305 (4.4141, -9.6545) -> (4.8, -9.8144) projected
  line L306 (4.8, -9.8144) -> (5.1314, -10.0686) projected
  line L307 (5.1314, -10.0686) -> (5.3856, -10.4) projected
  line L308 (5.3856, -10.4) -> (5.5455, -10.7859) projected
  line L309 (5.5455, -10.7859) -> (5.6, -11.2) projected
  line L310 (5.6, -11.2) -> (5.5455, -11.6141) projected
  line L311 (5.5455, -11.6141) -> (5.3856, -12) projected
  line L312 (-135.5455, -10.7859) -> (-135.3856, -10.4) projected
  line L313 (-135.3856, -10.4) -> (-135.1314, -10.0686) projected
  line L314 (-135.1314, -10.0686) -> (-134.8, -9.8144) projected
  line L315 (-134.8, -9.8144) -> (-134.4141, -9.6545) projected
  line L316 (-134.4141, -9.6545) -> (-134, -9.6) projected
  line L317 (-134, -9.6) -> (-133.5859, -9.6545) projected
  line L318 (-133.5859, -9.6545) -> (-133.2, -9.8144) projected
  line L319 (-133.2, -9.8144) -> (-132.8686, -10.0686) projected
  line L320 (-132.8686, -10.0686) -> (-132.6144, -10.4) projected
  line L321 (-132.6144, -10.4) -> (-132.4545, -10.7859) projected
  line L322 (-132.4545, -10.7859) -> (-132.4, -11.2) projected
  line L323 (-132.4, -11.2) -> (-132.4545, -11.6141) projected
  line L324 (-132.4545, -11.6141) -> (-132.6144, -12) projected
  line L325 (-132.6144, -12) -> (-132.8686, -12.3314) projected
  line L326 (-132.8686, -12.3314) -> (-133.2, -12.5856) projected
  line L327 (-133.2, -12.5856) -> (-133.5859, -12.7455) projected
  line L328 (-133.5859, -12.7455) -> (-134, -12.8) projected
  line L329 (-134, -12.8) -> (-134.4141, -12.7455) projected
  line L330 (-134.4141, -12.7455) -> (-134.8, -12.5856) projected
  line L331 (-134.8, -12.5856) -> (-135.1314, -12.3314) projected
  line L332 (-135.1314, -12.3314) -> (-135.3856, -12) projected
  line L333 (-135.3856, -12) -> (-135.5455, -11.6141) projected
  line L334 (-135.5455, -11.6141) -> (-135.6, -11.2) projected
  line L335 (-135.6, -11.2) -> (-135.5455, -10.7859) projected
  line L336 (11, 28.649) -> (11, 15.6085)
  line L337 (11, 28.649) -> (24.0405, 28.649) construction
  line L338 (11, 28.649) -> (5.8066, 28.8251)
  line L339 (5.8066, 28.8251) -> (5.2585, 12.6618)
  line L340 (5.2585, 12.6618) -> (16.8682, 15.0954)
  line L341 (16.8682, 15.0954) -> (15.2904, 19.2664)
  line L342 (11, 19.2664) -> (15.2904, 19.2664)
  line L343 (18, 19.2664) -> (12.5808, 19.2664)
  line L344 (8, 24.0664) -> (0.5711, 24.0664)
  point P0 (0, 0)
  dimension "d12" = 90
  dimension "d13" = 90
  constraints: 68 end point, 16 centre point, 11 point on circle, 3 point on line, 1 horizontal, 1 midpoint
  measures "d12" angle of L336 L337
  measures "d13" angle of L339 L338
extrude "Extrusion3" add sketch "Sketch3" against normal up to surface (6 mm away) contours L341 L340 L339 L344 A3 A2 A1 L336 L342 L0 | A1 A2 A3 A4 L336 | A4 A3 L344 L339 L338
fillet "Fillet6" radius 2 1 edges at (11, 20.0413, 3)
sketch "Sketch4" plane through (0, 0, 6) normal (0, 0, 1) x (1, 0, 0)
  circle A0 centre (0.9394, 23.7332) radius 5.8586
  point P0 (0, 0)
  constraints: 1 centre point
extrude "Extrusion4" cut sketch "Sketch4" against normal blind 10
fillet "Fillet7" radius 2 2 edges at (2.4, 18.0595, 3) (2.4, 29.4068, 3)